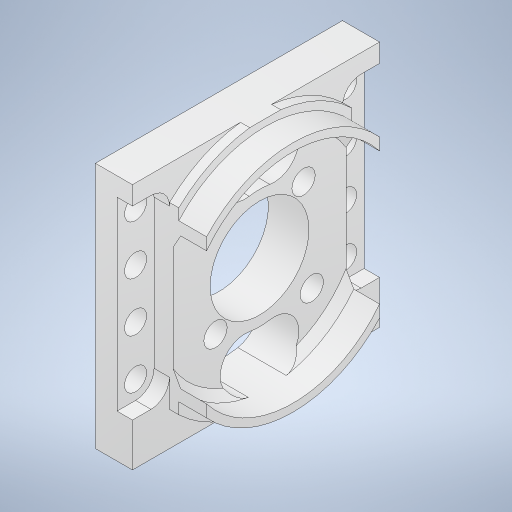
# Autodesk Inventor part: Motor Plate
Saved by Autodesk Inventor 2023.2 (Build 272271000, 271)
## iProperties
Created: 2024-02-17
Part Number: Motor Plate
Material: Aluminum 6061
Document SubType Name: Modeling
Designer: Nathan Cai
Density: 2.7 g/cm^3
Appearance: Aluminum - Flat
Mass: 9.38156 g
Surface Area: 33.2429 cm^2
Volume: 3.47465 cm^3
Author: Nathan Cai
Autodesk Inventor part; units mm, degrees
ref_plane "YZ Plane" through (0, 0, 0) normal (1, 0, 0) x (0, 1, 0)
ref_plane "XZ Plane" through (0, 0, 0) normal (0, 1, 0) x (-1, 0, 0)
ref_plane "XY Plane" through (0, 0, 0) normal (0, 0, 1) x (1, 0, 0)
sketch "Sketch4" plane through (0, 0, 0) normal (1, 0, 0) x (0, 1, 0)
  line L0 (15.875, 15.875) -> (-15.875, 15.875)
  line L1 (-15.875, 15.875) -> (-15.875, -15.875)
  line L2 (-15.875, -15.875) -> (15.875, -15.875)
  line L3 (15.875, -15.875) -> (15.875, 15.875)
  line L4 (15.875, 15.875) -> (-15.875, -15.875) construction
  line L5 (-15.875, 15.875) -> (15.875, -15.875) construction
  circle A0 centre (0, 0) radius 6.35
  line L6 (0, 0) -> (0, 15.875) construction
  line L7 (0, 22.4506) -> (-22.4506, 0)
  line L8 (-22.4506, 0) -> (0, -22.4506)
  line L9 (0, -22.4506) -> (22.4506, 0)
  line L10 (22.4506, 0) -> (0, 22.4506)
  line L11 (0, 22.4506) -> (0, -22.4506) construction
  line L12 (-22.4506, 0) -> (22.4506, 0) construction
  point P0 (15.875, 6.5756)
  point P1 (6.5756, 15.875)
  point P2 (-6.5756, 15.875)
  point P3 (-15.875, 6.5756)
  point P4 (-15.875, -6.5756)
  point P5 (-6.5756, -15.875)
  point P6 (6.5756, -15.875)
  point P7 (15.875, -6.5756)
  dimension "d37" = 31.75
  dimension "d38" = 31.75
  dimension "d39" = 12.7
  dimension "d126" = 31.75
  dimension "d127" = 31.75
  dimension "d128" = 45
  constraints: 26 end point, 4 midpoint, 4 parallel, 2 perpendicular, 1 centre point, 1 coincident, 1 horizontal
  measures "d37" distance of L2.end L1.end
  measures "d38" distance of L1.end L0.end
  measures "d39" diameter of A0
  measures "d126" distance between parallel lines of L7 L9
  measures "d127" distance between parallel lines of L10 L8
  measures "d128" angle of L12 L4
extrude "Extrusion5" add sketch "Sketch4" along normal blind 9.525 contours L3 L10 L0 | L10 L3 L9 L2 L8 L1 L7 L0 | L7 L1 L0 | L3 L2 L9 | L8 L2 L1
sketch "Sketch5" plane through (9.525, 0, 0) normal (1, 0, 0) x (0, 0, -1)
  circle A0 centre (0, 0) radius 25.4
  circle A1 centre (0, 0) radius 15
  circle A2 centre (0, 0) radius 14
  circle A3 centre (0, 0) radius 16
  dimension "d50" = 50.8
  dimension "d51" = 30
  dimension "d52" = 1
  dimension "d55" = 1
  constraints: 4 centre point, 2 coincident
  measures "d50" diameter of A0
  measures "d51" diameter of A1
  measures "d52" radial gap between concentric circles of A1 A2
  measures "d55" radial gap between concentric circles of A1 A3
extrude "Extrusion6" cut sketch "Sketch5" against normal blind 3.5719 contours A0 | A3
extrude "Extrusion7" cut sketch "Sketch5" against normal blind 4.7625 contours A0
sketch "Sketch7" plane through (9.525, 0, 0) normal (1, 0, 0) x (0, 0, -1)
  circle A0 centre (0, 0) radius 14
  circle A1 centre (0, 0) radius 15 projected
  dimension "d97" = 1
  constraints: 1 centre point, 1 coincident
  measures "d97" radial gap between concentric circles of A0 A1
extrude "Extrusion10" cut sketch "Sketch7" against normal blind 4.3094 contours A0
chamfer "Chamfer8" distance 1 angle 45 1 edges at (5.2156, 0, 14)
sketch "Sketch8" plane through (5.2156, 0, 0) normal (1, 0, 0) x (0, 0, -1)
  circle A0 centre (0, 0) radius 8 construction
  line L0 (0, 0) -> (8, 0) construction
  line L1 (0, 0) -> (5.6569, 5.6569) construction
  circle A1 centre (5.6569, 5.6569) radius 1.5
  circle A2 centre (0, 0) radius 9.5 construction
  line L2 (0, 0) -> (6.7175, -6.7175) construction
  circle A3 centre (6.7175, -6.7175) radius 1.5
  circle A4 centre (-6.7175, 6.7175) radius 1.5
  circle A5 centre (-5.6569, -5.6569) radius 1.5
  arc A6 (-1.8797, -10.6605) -> (1.8797, -10.6605) centre (0, 0) ccw construction
  arc A7 (-2.4311, -13.7873) -> (2.4311, -13.7873) centre (0, 0) ccw
  arc A8 (-1.3284, -7.5338) -> (1.3284, -7.5338) centre (0, 0) ccw
  arc A9 (-1.3284, -7.5338) -> (-2.4311, -13.7873) centre (-1.8797, -10.6605) ccw
  arc A10 (2.4311, -13.7873) -> (1.3284, -7.5338) centre (1.8797, -10.6605) ccw
  circle A11 centre (0, 0) radius 14 projected
  line L3 (0, -10.825) -> (0, 0) construction
  line L4 (1.8797, -10.6605) -> (0, 0) construction
  arc A12 (1.8797, 10.6605) -> (-1.8797, 10.6605) centre (0, 0) ccw construction
  arc A13 (-2.4311, 13.7873) -> (-1.3284, 7.5338) centre (-1.8797, 10.6605) ccw
  arc A14 (2.4311, 13.7873) -> (-2.4311, 13.7873) centre (0, 0) ccw
  arc A15 (1.3284, 7.5338) -> (2.4311, 13.7873) centre (1.8797, 10.6605) ccw
  arc A16 (1.3284, 7.5338) -> (-1.3284, 7.5338) centre (0, 0) ccw
  point P0 (0, 10.825)
  point P1 (2.4311, 13.7873)
  point P2 (-2.4311, 13.7873)
  dimension "d150" = 19
  dimension "d70" = 16
  dimension "d71" = 3
  dimension "d72" = 45
  dimension "d151" = 3
  dimension "d154" = 360
  dimension "d169" = 3.175
  dimension "d170" = 45
  dimension "d171" = 10
  dimension "d174" = 360
  constraints: 23 point on circle, 15 centre point, 10 end point, 4 coincident, 4 tangent, 1 horizontal, 1 perpendicular, 42 other
  measures "d70" diameter of A0
  measures "d71" diameter of A1
  measures "d72" angle of L0 L1
  measures "d151" diameter of A3
  measures "d169" radius of A9
  measures "d170" angle of L2 L3
  measures "d171" angle of L3 L4
extrude "Extrusion11" cut sketch "Sketch8" along normal through all both and the other way through all contours A1 | A3 | A4 | A5 | A9 A8 A10 A7 | A11 A15 A16 A13
sketch "Sketch14" plane through (9.525, 0, 0) normal (1, 0, 0) x (0, 0, -1)
  line L0 (15.875, -15.875) -> (15.875, 15.875) projected
  line L1 (-15.875, -15.875) -> (15.875, -15.875) projected
  line L2 (15.875, 15.875) -> (11.1125, 15.875)
  line L3 (11.1125, 15.875) -> (11.1125, -15.875)
  line L4 (11.1125, -15.875) -> (15.875, -15.875)
  line L5 (15.875, -15.875) -> (15.875, 15.875)
  line L6 (15.875, 15.875) -> (-15.875, 15.875) projected
  line L7 (-1.9961, -15.875) -> (-15.875, -15.875) projected
  line L8 (-15.875, 15.875) -> (-11.1125, 15.875)
  line L9 (-11.1125, 15.875) -> (-11.1125, -15.875)
  line L10 (-11.1125, -15.875) -> (-15.875, -15.875)
  line L11 (-15.875, -15.875) -> (-15.875, 15.875)
  point P0 (0, 0)
  point P1 (-11.1125, -15.875)
  dimension "d206" = 4.7625
  dimension "d207" = 4.7625
  constraints: 16 end point, 4 parallel, 2 horizontal, 2 perpendicular, 2 point on line
  measures "d206" distance of L4.end L3.end
  measures "d207" distance of L9.end L10.end
extrude "Extrusion17" cut sketch "Sketch14" against normal up to surface (4.7625 mm away) contours L1 L3 L2 L0 | L9 L1 L11 L6
sketch "Sketch15" plane through (9.525, 0, 0) normal (1, 0, 0) x (0, 0, -1)
  line L0 (15.875, -15.875) -> (15.875, 15.875) projected
  line L1 (15.875, 13.4938) -> (11.1125, 13.4938)
  line L2 (11.1125, 13.4938) -> (11.1125, -13.4938)
  line L3 (11.1125, -13.4938) -> (15.875, -13.4938)
  line L4 (15.875, -13.4938) -> (15.875, 13.4938)
  line L5 (-1.9961, 15.875) -> (1.9961, 15.875) projected
  line L6 (0, 15.875) -> (0, -15.875) construction
  line L7 (-15.875, -15.875) -> (15.875, -15.875) projected
  line L8 (13.4938, 13.4938) -> (13.4938, -13.4938) construction
  circle A0 centre (13.4938, 11.1125) radius 1.4224
  circle A1 centre (13.4938, 4.7625) radius 1.4224
  circle A2 centre (13.4938, -1.5875) radius 1.4224
  circle A3 centre (13.4938, -7.9375) radius 1.4224
  line L9 (15.875, 0) -> (11.1125, 0) construction
  line L10 (-15.875, 13.4938) -> (-11.1125, 13.4938)
  line L11 (-11.1125, 13.4938) -> (-11.1125, -13.4938)
  line L12 (-11.1125, -13.4938) -> (-15.875, -13.4938)
  line L13 (-15.875, -13.4938) -> (-15.875, 13.4938)
  line L14 (-13.4938, 13.4938) -> (-13.4938, -13.4938) construction
  circle A4 centre (-13.4938, 11.1125) radius 1.4224
  circle A5 centre (-13.4938, 4.7625) radius 1.4224
  circle A6 centre (-13.4938, -1.5875) radius 1.4224
  circle A7 centre (-13.4938, -7.9375) radius 1.4224
  line L15 (-15.875, 0) -> (-11.1125, 0) construction
  point P0 (0, 0)
  point P1 (0, 0)
  dimension "d210" = 4.7625
  dimension "d211" = 26.9875
  dimension "d212" = 2.8448
  dimension "d213" = 2.3813
  dimension "d216" = 6.35
  constraints: 26 end point, 12 symmetric about line, 8 centre point, 7 midpoint, 4 point on line, 2 parallel, 1 horizontal, 1 perpendicular, 1 vertical, 10 other
  measures "d210" distance of L3.end L2.end
  measures "d211" distance between parallel lines of L1 L3
  measures "d212" diameter of A0
  measures "d213" distance from line of L1 A0.centre
  measures "d216" distance of A0.centre A1.centre
extrude "Extrusion18" cut sketch "Sketch15" against normal through all contours A0 | A1 | A2 | A3 | A4 | A5 | A6 | A7
sketch "Sketch16" plane through (5.9531, 0, 0) normal (1, 0, 0) x (0, 0, -1)
  circle A0 centre (-13.4938, -1.5875) radius 1.4224 construction
  circle A1 centre (-13.4938, 4.7625) radius 1.4224 construction
  circle A2 centre (-13.4938, -7.9375) radius 1.4224 construction
  circle A3 centre (-13.4938, 11.1125) radius 1.4224 construction
  line L0 (-1.9961, -15.875) -> (-15.875, -15.875) construction
  arc A4 (-11.1125, -11.5114) -> (-1.9961, -15.875) centre (0, 0) ccw construction
  line L1 (-11.1125, 11.5114) -> (-11.1125, -11.5114) projected
  arc A5 (-1.9961, 15.875) -> (-11.1125, 11.5114) centre (0, 0) ccw construction
  line L2 (-15.875, 15.875) -> (-1.9961, 15.875) construction
  line L3 (-15.875, -15.875) -> (-15.875, 15.875) construction
  circle A6 centre (13.4938, 4.7625) radius 1.4224 construction
  circle A7 centre (13.4938, -1.5875) radius 1.4224 construction
  circle A8 centre (13.4938, 11.1125) radius 1.4224 construction
  circle A9 centre (13.4938, -7.9375) radius 1.4224 construction
  line L4 (1.9961, 15.875) -> (15.875, 15.875) construction
  arc A10 (11.1125, 11.5114) -> (1.9961, 15.875) centre (0, 0) ccw construction
  line L5 (11.1125, -11.5114) -> (11.1125, 11.5114) projected
  arc A11 (1.9961, -15.875) -> (11.1125, -11.5114) centre (0, 0) ccw construction
  line L6 (15.875, -15.875) -> (1.9961, -15.875) construction
  line L7 (15.875, 15.875) -> (15.875, -15.875) construction
  circle A12 centre (-13.4938, -7.9375) radius 2.3812
  circle A13 centre (-13.4938, -1.5875) radius 2.3812
  circle A14 centre (-13.4938, 4.7625) radius 2.3812
  circle A15 centre (-13.4938, 11.1125) radius 2.3812
  circle A16 centre (13.4938, -7.9375) radius 2.3812
  circle A17 centre (13.4938, -1.5875) radius 2.3812
  circle A18 centre (13.4938, 4.7625) radius 2.3812
  circle A19 centre (13.4938, 11.1125) radius 2.3812
  line L8 (15.875, 15.875) -> (15.875, -15.875) projected
  line L9 (13.4938, 13.4937) -> (15.875, 13.4937)
  line L10 (15.875, 13.4937) -> (15.875, -10.3188)
  line L11 (15.875, -10.3188) -> (13.4938, -10.3188)
  line L12 (13.4938, -10.3188) -> (13.4938, 13.4937) construction
  line L13 (-15.875, -15.875) -> (-15.875, 15.875) projected
  line L14 (-13.4938, 13.4937) -> (-15.875, 13.4937)
  line L15 (-15.875, 13.4937) -> (-15.875, -10.3188)
  line L16 (-15.875, -10.3188) -> (-13.4938, -10.3188)
  line L17 (-13.4938, -10.3188) -> (-13.4938, 13.4937) construction
  point P0 (-15.875, -7.9375)
  point P1 (-15.875, -1.5875)
  point P2 (-11.1125, -7.9375)
  point P3 (-11.1125, -1.5875)
  point P4 (-15.875, 4.7625)
  point P5 (-11.1125, 4.7625)
  point P6 (-15.875, 11.1125)
  point P7 (-11.1125, 11.1125)
  point P8 (15.875, -7.9375)
  point P9 (15.875, -1.5875)
  point P10 (11.1125, -1.5875)
  point P11 (11.1125, -7.9375)
  point P12 (15.875, 4.7625)
  point P13 (11.1125, 4.7625)
  point P14 (15.875, 11.1125)
  point P15 (11.1125, 11.1125)
  dimension "d223" = 4.7625
  dimension "d224" = 6.35
  dimension "d225" = 26.9875
  dimension "d228" = 6.35
  dimension "d231" = 26.9875
  constraints: 16 end point, 6 centre point, 6 horizontal, 4 parallel, 3 tangent, 2 perpendicular, 2 point on line, 1 coincident, 1 vertical, 18 other
  measures "d223" diameter of A12
  measures "d224" distance between centres of A2 A0
  measures "d225" distance of A9.centre A2.centre
  measures "d228" distance of A12.centre A13.centre
  measures "d231" distance of A12.centre A16.centre
extrude "Extrusion19" cut sketch "Sketch16" against normal blind 3.175
equation "\"d37\" = d38"
equation "\"d126\" = d37"
equation "\"d127\" = d126"
body "Solid2"
